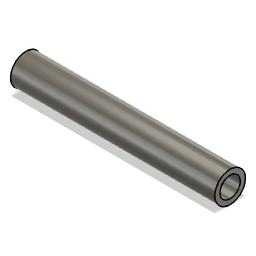
SwagelokTube v7 (Autodesk Fusion 360 design; units mm, degrees)
Autodesk Fusion 360 part; units mm, degrees
sketch "Skizze1" plane through (0, 0, 0) normal (1, 0, 0) x (0, 0, -1)
  circle A0 centre (0, 0) radius 3
  circle A1 centre (0, 0) radius 2
  dimension "d1" = 6
  dimension "d2" = 4
  constraint coincident A0.centre A1.centre
  measures "d1" diameter of A0
  measures "d2" diameter of A1
extrude "Extrusion1" add sketch "Skizze1" along normal blind 40 makes body 1
copy_body "Körper->Berechn1" bodies 1 removing the originals makes body 2 in component "SwagelokTube"
component "SwagelokTube" placed x (1, 0, 0) y (0, 1, 0) z (0, 0, 1) at (0, 0, 0)
